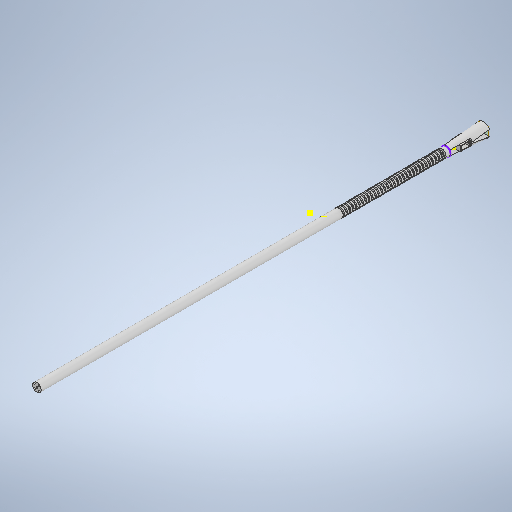
# Autodesk Inventor part: Tool 1
Saved by Autodesk Inventor 2025.2 (Build 292293000, 293)
## iProperties
Created: 2025-03-11
Part Number: Tool 1
Material: Generic
Document SubType Name: Modeling
Designer: avnr2
Density: 1 g/cm^3
Appearance: Default
Author: avnr2
Autodesk Inventor part; units mm, degrees
sketch "Sketch1" plane through (0, 0, 0) normal (0, 1, 0) x (-1, 0, 0)
  circle A0 centre (0, 0) radius 1.5
  dimension "d0" = 3
  constraints: 1 centre point, 1 coincident
  measures "d0" diameter of A0
extrude "Extrusion1" add sketch "Sketch1" along normal blind 40
ref_plane "Work Plane1" through (-40, 0, 0) normal (1, 0, 0) x (0, 1, 0)
sketch "Sketch2" plane through (-40, 0, 0) normal (1, 0, 0) x (0, 1, 0)
  line L0 (0, -1.5) -> (40, -1.5) projected
  line L1 (39.7, -1.5) -> (39.2, -1.5)
  line L2 (39.2, -1.5) -> (39.2, -0.2)
  line L3 (39.2, -0.2) -> (39.7, -0.2)
  line L4 (39.7, -0.2) -> (39.7, -1.5)
  line L5 (38.6, -1.5) -> (38.1, -1.5)
  line L6 (38.1, -1.5) -> (38.1, -0.2)
  line L7 (38.1, -0.2) -> (38.6, -0.2)
  line L8 (38.6, -0.2) -> (38.6, -1.5)
  line L9 (40, -1.5) -> (40, 1.5) projected
  line L10 (40, 0) -> (0, 0)
  line L11 (39.7, 1.5) -> (39.2, 1.5)
  line L12 (39.2, 1.5) -> (39.2, 0.2)
  line L13 (39.2, 0.2) -> (39.7, 0.2)
  line L14 (39.7, 0.2) -> (39.7, 1.5)
  line L15 (38.6, 1.5) -> (38.1, 1.5)
  line L16 (38.1, 1.5) -> (38.1, 0.2)
  line L17 (38.1, 0.2) -> (38.6, 0.2)
  line L18 (38.6, 0.2) -> (38.6, 1.5)
  line L19 (37.8, -1.5) -> (37.8, 1.5)
  line L20 (0, 1.5) -> (40, 1.5) projected
  line L21 (35.9, -1.5) -> (36.4, -1.5)
  line L22 (36.4, -1.5) -> (36.4, -0.2)
  line L23 (36.4, -0.2) -> (35.9, -0.2)
  line L24 (35.9, -0.2) -> (35.9, -1.5)
  line L25 (37, -1.5) -> (37.5, -1.5)
  line L26 (37.5, -1.5) -> (37.5, -0.2)
  line L27 (37.5, -0.2) -> (37, -0.2)
  line L28 (37, -0.2) -> (37, -1.5)
  line L29 (35.9, 1.5) -> (36.4, 1.5)
  line L30 (36.4, 1.5) -> (36.4, 0.2)
  line L31 (36.4, 0.2) -> (35.9, 0.2)
  line L32 (35.9, 0.2) -> (35.9, 1.5)
  line L33 (37, 1.5) -> (37.5, 1.5)
  line L34 (37.5, 1.5) -> (37.5, 0.2)
  line L35 (37.5, 0.2) -> (37, 0.2)
  line L36 (37, 0.2) -> (37, 1.5)
  line L37 (35.6, 1.5) -> (35.6, -1.5)
  line L38 (31.5, -1.5) -> (32, -1.5)
  line L39 (32, -1.5) -> (32, -0.2)
  line L40 (32, -0.2) -> (31.5, -0.2)
  line L41 (31.5, -0.2) -> (31.5, -1.5)
  line L42 (32.6, -1.5) -> (33.1, -1.5)
  line L43 (33.1, -1.5) -> (33.1, -0.2)
  line L44 (33.1, -0.2) -> (32.6, -0.2)
  line L45 (32.6, -0.2) -> (32.6, -1.5)
  line L46 (31.5, 1.5) -> (32, 1.5)
  line L47 (32, 1.5) -> (32, 0.2)
  line L48 (32, 0.2) -> (31.5, 0.2)
  line L49 (31.5, 0.2) -> (31.5, 1.5)
  line L50 (32.6, 1.5) -> (33.1, 1.5)
  line L51 (33.1, 1.5) -> (33.1, 0.2)
  line L52 (33.1, 0.2) -> (32.6, 0.2)
  line L53 (32.6, 0.2) -> (32.6, 1.5)
  line L54 (33.4, -1.5) -> (33.4, 1.5)
  line L55 (35.3, -1.5) -> (34.8, -1.5)
  line L56 (35.3, -0.2) -> (35.3, -1.5)
  line L57 (34.8, -1.5) -> (34.8, -0.2)
  line L58 (34.2, -1.5) -> (33.7, -1.5)
  line L59 (34.2, -0.2) -> (34.2, -1.5)
  line L60 (33.7, -1.5) -> (33.7, -0.2)
  line L61 (33.7, -0.2) -> (34.2, -0.2)
  line L62 (33.7, 0.2) -> (34.2, 0.2)
  line L63 (35.3, 0.2) -> (35.3, 1.5)
  line L64 (34.2, 0.2) -> (34.2, 1.5)
  line L65 (33.7, 1.5) -> (33.7, 0.2)
  line L66 (34.2, 1.5) -> (33.7, 1.5)
  line L67 (34.8, 1.5) -> (34.8, 0.2)
  line L68 (34.8, 0.2) -> (35.3, 0.2)
  line L69 (34.8, -0.2) -> (35.3, -0.2)
  line L70 (35.3, 1.5) -> (34.8, 1.5)
  line L71 (31.2, 1.5) -> (31.2, -1.5)
  line L72 (22.7, -1.5) -> (23.2, -1.5)
  line L73 (23.2, -1.5) -> (23.2, -0.2)
  line L74 (23.2, -0.2) -> (22.7, -0.2)
  line L75 (22.7, -0.2) -> (22.7, -1.5)
  line L76 (23.8, -1.5) -> (24.3, -1.5)
  line L77 (24.3, -1.5) -> (24.3, -0.2)
  line L78 (24.3, -0.2) -> (23.8, -0.2)
  line L79 (23.8, -0.2) -> (23.8, -1.5)
  line L80 (22.4, -1.5) -> (22.4, 1.5)
  line L81 (22.7, 1.5) -> (23.2, 1.5)
  line L82 (23.2, 1.5) -> (23.2, 0.2)
  line L83 (23.2, 0.2) -> (22.7, 0.2)
  line L84 (22.7, 0.2) -> (22.7, 1.5)
  line L85 (23.8, 1.5) -> (24.3, 1.5)
  line L86 (24.3, 1.5) -> (24.3, 0.2)
  line L87 (24.3, 0.2) -> (23.8, 0.2)
  line L88 (23.8, 0.2) -> (23.8, 1.5)
  line L89 (24.6, -1.5) -> (24.6, 1.5)
  line L90 (26.5, -1.5) -> (26, -1.5)
  line L91 (26.5, -0.2) -> (26.5, -1.5)
  line L92 (26, -1.5) -> (26, -0.2)
  line L93 (25.4, -1.5) -> (24.9, -1.5)
  line L94 (25.4, -0.2) -> (25.4, -1.5)
  line L95 (24.9, -1.5) -> (24.9, -0.2)
  line L96 (24.9, -0.2) -> (25.4, -0.2)
  line L97 (24.9, 0.2) -> (25.4, 0.2)
  line L98 (26.5, 0.2) -> (26.5, 1.5)
  line L99 (25.4, 0.2) -> (25.4, 1.5)
  line L100 (24.9, 1.5) -> (24.9, 0.2)
  line L101 (25.4, 1.5) -> (24.9, 1.5)
  line L102 (26, 1.5) -> (26, 0.2)
  line L103 (26, 0.2) -> (26.5, 0.2)
  line L104 (26, -0.2) -> (26.5, -0.2)
  line L105 (26.5, 1.5) -> (26, 1.5)
  line L106 (26.8, 1.5) -> (26.8, -1.5)
  line L107 (30.9, -1.5) -> (30.4, -1.5)
  line L108 (29.3, -1.5) -> (29.3, -0.2)
  line L109 (29.8, -1.5) -> (29.3, -1.5)
  line L110 (29.8, -0.2) -> (29.8, -1.5)
  line L111 (30.4, -1.5) -> (30.4, -0.2)
  line L112 (30.9, -0.2) -> (30.9, -1.5)
  line L113 (29.3, 1.5) -> (29.3, 0.2)
  line L114 (29.3, -0.2) -> (29.8, -0.2)
  line L115 (30.9, 1.5) -> (30.4, 1.5)
  line L116 (30.4, 0.2) -> (30.9, 0.2)
  line L117 (30.4, -0.2) -> (30.9, -0.2)
  line L118 (29, -1.5) -> (29, 1.5)
  line L119 (28.7, 1.5) -> (28.7, 0.2)
  line L120 (28.2, 0.2) -> (28.2, 1.5)
  line L121 (28.7, 0.2) -> (28.2, 0.2)
  line L122 (27.6, 1.5) -> (27.6, 0.2)
  line L123 (27.1, 0.2) -> (27.1, 1.5)
  line L124 (27.6, 0.2) -> (27.1, 0.2)
  line L125 (27.1, 1.5) -> (27.6, 1.5)
  line L126 (28.2, 1.5) -> (28.7, 1.5)
  line L127 (30.9, 0.2) -> (30.9, 1.5)
  line L128 (30.4, 1.5) -> (30.4, 0.2)
  line L129 (29.8, 1.5) -> (29.3, 1.5)
  line L130 (29.3, 0.2) -> (29.8, 0.2)
  line L131 (29.8, 0.2) -> (29.8, 1.5)
  line L132 (27.6, -0.2) -> (27.1, -0.2)
  line L133 (28.7, -0.2) -> (28.2, -0.2)
  line L134 (27.1, -1.5) -> (27.6, -1.5)
  line L135 (27.1, -0.2) -> (27.1, -1.5)
  line L136 (27.6, -1.5) -> (27.6, -0.2)
  line L137 (28.2, -0.2) -> (28.2, -1.5)
  line L138 (28.7, -1.5) -> (28.7, -0.2)
  line L139 (28.2, -1.5) -> (28.7, -1.5)
  line L140 (5.1, -1.5) -> (5.6, -1.5)
  line L141 (5.6, -1.5) -> (5.6, -0.2)
  line L142 (5.6, -0.2) -> (5.1, -0.2)
  line L143 (5.1, -0.2) -> (5.1, -1.5)
  line L144 (6.2, -1.5) -> (6.7, -1.5)
  line L145 (6.7, -1.5) -> (6.7, -0.2)
  line L146 (6.7, -0.2) -> (6.2, -0.2)
  line L147 (6.2, -0.2) -> (6.2, -1.5)
  line L148 (4.8, -1.5) -> (4.8, 1.5)
  line L149 (5.1, 1.5) -> (5.6, 1.5)
  line L150 (5.6, 1.5) -> (5.6, 0.2)
  line L151 (5.6, 0.2) -> (5.1, 0.2)
  line L152 (5.1, 0.2) -> (5.1, 1.5)
  line L153 (6.2, 1.5) -> (6.7, 1.5)
  line L154 (6.7, 1.5) -> (6.7, 0.2)
  line L155 (6.7, 0.2) -> (6.2, 0.2)
  line L156 (6.2, 0.2) -> (6.2, 1.5)
  line L157 (7, -1.5) -> (7, 1.5)
  line L158 (8.9, -1.5) -> (8.4, -1.5)
  line L159 (8.9, -0.2) -> (8.9, -1.5)
  line L160 (8.4, -1.5) -> (8.4, -0.2)
  line L161 (7.8, -1.5) -> (7.3, -1.5)
  line L162 (7.8, -0.2) -> (7.8, -1.5)
  line L163 (7.3, -1.5) -> (7.3, -0.2)
  line L164 (7.3, -0.2) -> (7.8, -0.2)
  line L165 (7.3, 0.2) -> (7.8, 0.2)
  line L166 (8.9, 0.2) -> (8.9, 1.5)
  line L167 (7.8, 0.2) -> (7.8, 1.5)
  line L168 (7.3, 1.5) -> (7.3, 0.2)
  line L169 (7.8, 1.5) -> (7.3, 1.5)
  line L170 (8.4, 1.5) -> (8.4, 0.2)
  line L171 (8.4, 0.2) -> (8.9, 0.2)
  line L172 (8.4, -0.2) -> (8.9, -0.2)
  line L173 (8.9, 1.5) -> (8.4, 1.5)
  line L174 (9.2, 1.5) -> (9.2, -1.5)
  line L175 (13.3, -1.5) -> (12.8, -1.5)
  line L176 (11.7, -1.5) -> (11.7, -0.2)
  line L177 (12.2, -1.5) -> (11.7, -1.5)
  line L178 (12.2, -0.2) -> (12.2, -1.5)
  line L179 (12.8, -1.5) -> (12.8, -0.2)
  line L180 (13.3, -0.2) -> (13.3, -1.5)
  line L181 (11.7, 1.5) -> (11.7, 0.2)
  line L182 (11.7, -0.2) -> (12.2, -0.2)
  line L183 (13.3, 1.5) -> (12.8, 1.5)
  line L184 (12.8, 0.2) -> (13.3, 0.2)
  line L185 (12.8, -0.2) -> (13.3, -0.2)
  line L186 (11.4, -1.5) -> (11.4, 1.5)
  line L187 (11.1, 1.5) -> (11.1, 0.2)
  line L188 (10.6, 0.2) -> (10.6, 1.5)
  line L189 (11.1, 0.2) -> (10.6, 0.2)
  line L190 (10, 1.5) -> (10, 0.2)
  line L191 (9.5, 0.2) -> (9.5, 1.5)
  line L192 (10, 0.2) -> (9.5, 0.2)
  line L193 (9.5, 1.5) -> (10, 1.5)
  line L194 (10.6, 1.5) -> (11.1, 1.5)
  line L195 (13.3, 0.2) -> (13.3, 1.5)
  line L196 (12.8, 1.5) -> (12.8, 0.2)
  line L197 (12.2, 1.5) -> (11.7, 1.5)
  line L198 (11.7, 0.2) -> (12.2, 0.2)
  line L199 (12.2, 0.2) -> (12.2, 1.5)
  line L200 (10, -0.2) -> (9.5, -0.2)
  line L201 (11.1, -0.2) -> (10.6, -0.2)
  line L202 (9.5, -1.5) -> (10, -1.5)
  line L203 (9.5, -0.2) -> (9.5, -1.5)
  line L204 (10, -1.5) -> (10, -0.2)
  line L205 (10.6, -0.2) -> (10.6, -1.5)
  line L206 (11.1, -1.5) -> (11.1, -0.2)
  line L207 (10.6, -1.5) -> (11.1, -1.5)
  line L208 (13.6, 1.5) -> (13.6, -1.5)
  line L209 (21.6, -0.2) -> (22.1, -0.2)
  line L210 (20.5, -0.2) -> (21, -0.2)
  line L211 (22.1, 1.5) -> (21.6, 1.5)
  line L212 (22.1, -1.5) -> (21.6, -1.5)
  line L213 (21.6, -1.5) -> (21.6, -0.2)
  line L214 (22.1, -0.2) -> (22.1, -1.5)
  line L215 (21, -0.2) -> (21, -1.5)
  line L216 (20.5, -1.5) -> (20.5, -0.2)
  line L217 (21, -1.5) -> (20.5, -1.5)
  line L218 (15.8, -1.5) -> (15.8, 1.5)
  line L219 (15, 0.2) -> (15, 1.5)
  line L220 (15, 1.5) -> (15.5, 1.5)
  line L221 (15.5, 0.2) -> (15, 0.2)
  line L222 (14.4, 1.5) -> (14.4, 0.2)
  line L223 (13.9, 0.2) -> (13.9, 1.5)
  line L224 (13.9, 1.5) -> (14.4, 1.5)
  line L225 (14.4, 0.2) -> (13.9, 0.2)
  line L226 (15.5, 1.5) -> (15.5, 0.2)
  line L227 (20.2, -1.5) -> (20.2, 1.5)
  line L228 (20.5, 1.5) -> (20.5, 0.2)
  line L229 (21, 1.5) -> (20.5, 1.5)
  line L230 (20.5, 0.2) -> (21, 0.2)
  line L231 (21, 0.2) -> (21, 1.5)
  line L232 (22.1, 0.2) -> (22.1, 1.5)
  line L233 (21.6, 0.2) -> (22.1, 0.2)
  line L234 (21.6, 1.5) -> (21.6, 0.2)
  line L235 (19.9, 1.5) -> (19.9, 0.2)
  line L236 (19.9, 0.2) -> (19.4, 0.2)
  line L237 (19.4, 0.2) -> (19.4, 1.5)
  line L238 (18.3, 1.5) -> (18.8, 1.5)
  line L239 (18.8, 1.5) -> (18.8, 0.2)
  line L240 (19.9, -0.2) -> (19.4, -0.2)
  line L241 (18.3, 0.2) -> (18.3, 1.5)
  line L242 (18.8, 0.2) -> (18.3, 0.2)
  line L243 (18, 1.5) -> (18, -1.5)
  line L244 (18.8, -0.2) -> (18.3, -0.2)
  line L245 (18.3, -1.5) -> (18.8, -1.5)
  line L246 (18.3, -0.2) -> (18.3, -1.5)
  line L247 (18.8, -1.5) -> (18.8, -0.2)
  line L248 (19.4, -0.2) -> (19.4, -1.5)
  line L249 (19.4, -1.5) -> (19.9, -1.5)
  line L250 (19.9, -1.5) -> (19.9, -0.2)
  line L251 (19.4, 1.5) -> (19.9, 1.5)
  line L252 (13.9, -1.5) -> (14.4, -1.5)
  line L253 (14.4, -0.2) -> (13.9, -0.2)
  line L254 (15.5, -0.2) -> (15, -0.2)
  line L255 (15.5, -1.5) -> (15.5, -0.2)
  line L256 (15, -1.5) -> (15.5, -1.5)
  line L257 (15, -0.2) -> (15, -1.5)
  line L258 (14.4, -1.5) -> (14.4, -0.2)
  line L259 (13.9, -0.2) -> (13.9, -1.5)
  line L260 (17.2, 0.2) -> (17.7, 0.2)
  line L261 (17.7, 0.2) -> (17.7, 1.5)
  line L262 (17.7, 1.5) -> (17.2, 1.5)
  line L263 (17.2, 1.5) -> (17.2, 0.2)
  line L264 (16.6, 0.2) -> (16.6, 1.5)
  line L265 (16.1, 1.5) -> (16.1, 0.2)
  line L266 (16.6, 1.5) -> (16.1, 1.5)
  line L267 (16.1, 0.2) -> (16.6, 0.2)
  line L268 (17.2, -0.2) -> (17.7, -0.2)
  line L269 (17.7, -0.2) -> (17.7, -1.5)
  line L270 (17.7, -1.5) -> (17.2, -1.5)
  line L271 (17.2, -1.5) -> (17.2, -0.2)
  line L272 (16.1, -0.2) -> (16.6, -0.2)
  line L273 (16.1, -1.5) -> (16.1, -0.2)
  line L274 (16.6, -1.5) -> (16.1, -1.5)
  line L275 (16.6, -0.2) -> (16.6, -1.5)
  point P0 (22.4, 0)
  point P1 (4.8, 0)
  dimension "d4" = 1.3
  dimension "d5" = 0.5
  dimension "d6" = 0.5
  dimension "d7" = 0.6
  dimension "d8" = 40
  dimension "d9" = 0.3
  dimension "d10" = 0.3
  dimension "d11" = 0.3
  dimension "d12" = 0.3
  constraints: 546 end point, 278 symmetric about line, 4 parallel, 3 perpendicular, 3 vertical, 2 horizontal, 1 midpoint, 10 other
  measures "d4" distance of L3.end L1.start
  measures "d5" distance of L2.end L3.end
  measures "d6" distance of L6.end L7.end
  measures "d7" distance between parallel lines of L8 L2
  measures "d8" distance of L10.start L10.end
  measures "d9" distance between parallel lines of L19 L6
  measures "d10" distance between parallel lines of L37 L24
  measures "d11" distance between parallel lines of L41 L71
  measures "d12" distance between parallel lines of L75 L80
extrude "Extrusion2" cut sketch "Sketch2" along normal blind 54.75 and the other way blind 5 contours L143 L142 L141 L0 | L147 L146 L145 L0 | L20 L150 L151 L152 | L163 L164 L162 L0 | L154 L155 L156 L20 | L20 L167 L165 L168 | L166 L171 L170 L20 | L20 L190 L192 L191 | L0 L160 L172 L159 | L203 L200 L204 L0 | L0 L205 L201 L206 | L176 L182 L178 L0 | L187 L189 L188 L20 | L20 L199 L198 L181 | L195 L184 L196 L20 | L20 L222 L225 L223 | L0 L179 L185 L180 | L259 L253 L258 L0 | L0 L257 L254 L255 | L273 L272 L275 L0 | L226 L221 L219 L20 | L20 L264 L267 L265 | L261 L260 L263 L20 | L20 L239 L242 L241 | L0 L271 L268 L269 | L246 L244 L247 L0 | L0 L248 L240 L250 | L216 L210 L215 L0 | L235 L236 L237 L20 | L20 L231 L230 L228 | L0 L213 L209 L214 | L75 L74 L73 L0 | L232 L233 L234 L20 | L20 L82 L83 L84 | L0 L79 L78 L77 | L95 L96 L94 L0 | L86 L87 L88 L20 | L20 L99 L97 L100 | L98 L103 L102 L20 | L20 L122 L124 L123 | L0 L92 L104 L91 | L135 L132 L136 L0 | L0 L137 L133 L138 | L108 L114 L110 L0 | L119 L121 L120 L20 | L20 L131 L130 L113 | L127 L116 L128 L20 | L20 L47 L48 L49 | L0 L111 L117 L112 | L41 L40 L39 L0 | L0 L45 L44 L43 | L60 L61 L59 L0 | L51 L52 L53 L20 | L20 L64 L62 L65 | L63 L68 L67 L20 | L20 L30 L31 L32 | L0 L57 L69 L56 | L24 L23 L22 L0 | L0 L28 L27 L26 | L6 L7 L8 L0 | L34 L35 L36 L20 | L15 L18 L17 L16 | L0 L2 L3 L4 | L14 L13 L12 L11
sketch "Sketch3" plane through (0, 0, 0) normal (0, -1, 0) x (1, 0, 0)
  circle A0 centre (0, 0) radius 0.3
  dimension "d17" = 0.6
  constraints: 1 centre point, 1 coincident
  measures "d17" diameter of A0
extrude "Extrusion3" cut sketch "Sketch3" against normal blind 54.75
sketch "Sketch4" plane through (0, 0, 0) normal (0, -1, 0) x (1, 0, 0)
  circle A0 centre (0, 0) radius 1.15 construction
  circle A1 centre (-0.7909, -0.8348) radius 0.3
  circle A2 centre (0, 0) radius 1.15 construction
  circle A3 centre (0.8348, -0.7909) radius 0.3
  circle A4 centre (0, 0) radius 1.15 construction
  circle A5 centre (0.7909, 0.8348) radius 0.3
  circle A6 centre (0, 0) radius 1.15 construction
  circle A7 centre (-0.8348, 0.7909) radius 0.3
  dimension "d23" = 2.3
  dimension "d22" = 0.6
  dimension "d26" = 360
  constraints: 6 coincident, 4 centre point, 31 other
  measures "d22" diameter of A1
extrude "Extrusion4" cut sketch "Sketch4" against normal blind 54.75
sketch "Sketch5" plane through (0, 40, 0) normal (0, 1, 0) x (1, 0, 0)
  point P0 (0, 0)
sketch "Sketch6" plane through (0, 40, 0) normal (0, 1, 0) x (1, 0, 0)
  circle A0 centre (0, 0) radius 0.3 projected
  circle A1 centre (0, 0) radius 0.7513
  constraints: 1 centre point, 1 coincident
extrude "Extrusion5" add sketch "Sketch6" along normal blind 0.6
sketch "Sketch7" plane through (0, 40.6, 0) normal (0, 1, 0) x (1, 0, 0)
  circle A0 centre (0, 0) radius 1.5
  constraints: 1 centre point, 1 coincident
extrude "Extrusion6" add sketch "Sketch7" along normal blind 0.6
sketch "Sketch8" plane through (0, 41.2, 0) normal (0, 1, 0) x (1, 0, 0)
  circle A0 centre (0, 0) radius 0.3 projected
  circle A1 centre (0, 0) radius 0.3
  constraints: 1 centre point, 1 coincident
extrude "Extrusion7" cut sketch "Sketch8" against normal blind 0.6
sketch "Sketch9" plane through (0, 41.2, 0) normal (0, 1, 0) x (1, 0, 0)
  circle A0 centre (0, 0) radius 1.5
  constraints: 1 centre point, 1 coincident
extrude "Extrusion8" add sketch "Sketch9" along normal blind 10
ref_plane "Work Plane2" through (-13.25, 0, 0) normal (1, 0, 0) x (0, 1, 0)
sketch "Sketch10" plane through (-13.25, 0, 0) normal (1, 0, 0) x (0, 1, 0)
  line L0 (51.2, -1.5) -> (51.2, 1.5) projected
  line L1 (51.2, 0) -> (42.026, 0)
  line L2 (51.2, 0.05) -> (47.2, 0.05)
  line L3 (47.2, 0.05) -> (47.2, -0.05)
  line L4 (47.2, -0.05) -> (51.2, -0.05)
  line L5 (51.2, -0.05) -> (51.2, 0.05)
  line L6 (51.2, 0.05) -> (47.2, -0.05) construction
  line L7 (47.2, 0.05) -> (51.2, -0.05) construction
  point P0 (0, 0)
  point P1 (49.2, 0)
  dimension "d39" = 4
  dimension "d40" = 0.1
  constraints: 14 end point, 4 midpoint, 2 horizontal, 2 parallel, 1 perpendicular, 1 point on line
  measures "d39" distance of L3.end L4.end
  measures "d40" distance of L2.end L3.end
extrude "Extrusion9" cut sketch "Sketch10" along normal blind 20.75
sketch "Sketch11" plane through (-13.25, 0, 0) normal (1, 0, 0) x (0, 1, 0)
  line L0 (47.2, 0.05) -> (51.2, 0.05) projected
  line L1 (47.2, 0.05) -> (47, 0.05)
  line L2 (47, 0.05) -> (47, 0.55)
  line L3 (47, 0.55) -> (45, 0.55)
  line L4 (45, -0.5) -> (47, -0.5)
  line L5 (47, -0.5) -> (47, -0.05)
  line L6 (47.2, -0.05) -> (51.2, -0.05) projected
  line L7 (47, -0.05) -> (47.2, -0.05)
  line L8 (47.2, -0.05) -> (47.2, -0.3)
  line L9 (47.2, -0.3) -> (47.1, -0.3)
  line L10 (47.1, -0.3) -> (47.1, -0.7)
  line L11 (47.1, -0.7) -> (44.6, -0.7)
  line L12 (44.6, 0.75) -> (47.1, 0.75)
  line L13 (47.1, 0.75) -> (47.1, 0.3)
  line L14 (47.1, 0.3) -> (47.2, 0.3)
  line L15 (47.2, 0.3) -> (47.2, 0.05)
  line L16 (47.2, 0.05) -> (47.2, -0.05) projected
  line L17 (47.2, 0) -> (44.6089, 0)
  line L18 (45, 0.55) -> (45, -0.5)
  line L19 (44.6, 0.75) -> (44.6, -0.7)
  line L20 (47.2, 0.3) -> (47.2, 1)
  line L21 (47.2, 1) -> (41.9867, 1)
  line L22 (47.2, -0.3) -> (47.2, -1)
  line L23 (47.2, -1) -> (41.9867, -1)
  line L24 (40.6, -1.5) -> (51.2, -1.5) projected
  line L25 (41.9867, -1) -> (41.9867, 1)
  point P0 (0, 0)
  dimension "d43" = 0.2
  dimension "d44" = 0.5
  dimension "d45" = 2
  dimension "d48" = 0.25
  dimension "d51" = 0.75
  dimension "d52" = 0.2
  dimension "d53" = 0.2
  dimension "d54" = 2.5911
  dimension "d55" = 0.5
  dimension "d56" = 0.1
  dimension "d57" = 0.2
  dimension "d58" = 0.25
  dimension "d59" = 2.5
  dimension "d60" = 2.5
  dimension "d67" = 1
  dimension "d68" = 1
  constraints: 44 end point, 11 perpendicular, 6 horizontal alignment, 6 vertical alignment, 4 point on line, 3 parallel, 2 horizontal, 2 vertical, 1 midpoint
  measures "d43" distance of L0.start L1.end
  measures "d44" distance of L1.end L2.end
  measures "d45" distance of L2.end L3.end
  measures "d48" distance of L14.end L0.start
  measures "d51" distance between parallel lines of L17 L12
  measures "d52" distance between parallel lines of L3 L12
  measures "d53" distance between parallel lines of L11 L4
  measures "d54" distance of L17.start L17.end
  measures "d55" distance between parallel lines of L4 L17
  measures "d56" distance of L8.end L9.end
  measures "d57" distance between parallel lines of L5 L8
  measures "d58" distance between parallel lines of L9 L7
  measures "d59" distance of L10.end L11.end
  measures "d60" distance of L12.start L12.end
  measures "d67" distance between parallel lines of L17 L21
  measures "d68" distance between parallel lines of L17 L23
extrude "Extrusion10" cut sketch "Sketch11" along normal blind 20.754 contours L16 L17 L18 L3 L2 L1 | L14 L13 L12 L19 L11 L10 L9 L22 L23 L25 L21 L20 | L16 L7 L5 L4 L18 L17
sketch "Sketch12" plane through (-1.3266, 44.6, -0.7) normal (0, -1, 0) x (1, 0, 0)
  point P0 (1.3266, 0.7)
sketch "Sketch13" plane through (-1.118, 41.9867, 1) normal (0, 1, 0) x (1, 0, 0)
  point P0 (1.118, 1)
sketch "Sketch14" plane through (0, 0, 0) normal (0, -1, 0) x (1, 0, 0)
  circle A0 centre (0, 0) radius 0.3
  constraints: 1 centre point, 1 coincident
extrude "Extrusion11" cut sketch "Sketch14" against normal blind 46.004
sketch "Sketch16" plane through (-1.299, 44.6, 0.75) normal (0, 0, 1) x (1, 0, 0)
  point P0 (1.299, -44.6)
sketch "Sketch17" plane through (0, 40.6, 0) normal (0, -1, 0) x (1, 0, 0)
  circle A0 centre (0, 0) radius 0.3
  circle A1 centre (0.8348, -0.7909) radius 0.3 projected
  circle A2 centre (0.8348, -0.7909) radius 0.3
  circle A3 centre (-0.7909, -0.8348) radius 0.3 projected
  circle A4 centre (-0.7909, -0.8348) radius 0.3
  circle A5 centre (-0.8348, 0.7909) radius 0.3 projected
  circle A6 centre (-0.8348, 0.7909) radius 0.3
  circle A7 centre (0.7909, 0.8348) radius 0.3 projected
  circle A8 centre (0.7909, 0.8348) radius 0.3
  circle A9 centre (0, 0) radius 0.3
  circle A10 centre (0, 0) radius 1.5
  constraints: 7 centre point, 7 coincident, 1 concentric
sketch "Sketch18" plane through (0, 0, 0) normal (0, -1, 0) x (1, 0, 0)
  point P0 (0, 0)
sketch "Sketch19" plane through (0, 0, 0) normal (0, -1, 0) x (1, 0, 0)
  arc A0 (-0.2236, -0.2) -> (0.2236, -0.2) centre (0, 0) ccw projected
  circle A1 centre (0, 0) radius 0.3
  circle A2 centre (-0.7892, -0.8405) radius 0.2991
  circle A3 centre (-0.8354, 0.7848) radius 0.2954
  circle A4 centre (0.7909, 0.8348) radius 0.3 projected
  circle A5 centre (0.7909, 0.8348) radius 0.3
  circle A6 centre (0.8348, -0.7909) radius 0.3 projected
  circle A7 centre (0.8348, -0.7909) radius 0.3
  circle A8 centre (0, 0) radius 1.5
  constraints: 6 centre point, 4 coincident
extrude "Extrusion13" add sketch "Sketch19" along normal blind 99
sketch "Sketch21" plane through (0, 51.2, 0) normal (0, 1, 0) x (1, 0, 0)
  circle A0 centre (0, 0) radius 1.5
  constraints: 1 centre point, 1 coincident
extrude "Extrusion14" cut sketch "Sketch21" against normal blind 4
extrude "Extrusion18" cut sketch "Sketch17" against normal blind 8 contours A0 | A1 | A3 | A5 | A7 | A10
sketch "Sketch36" plane through (0, 40.6, 0) normal (0, 1, 0) x (1, 0, 0)
  circle A0 centre (0, 0) radius 1.5
  constraints: 1 centre point, 1 coincident
extrude "Extrusion19" add sketch "Sketch36" along normal blind 1.5
sketch "Sketch37" plane through (0, 42.1, 0) normal (0, 1, 0) x (1, 0, 0)
  circle A0 centre (0, 0) radius 0.3
  dimension "d97" = 0.6
  constraints: 1 centre point, 1 coincident
  measures "d97" diameter of A0
extrude "Extrusion20" cut sketch "Sketch37" against normal blind 1.5
ref_plane "Work Plane3" through (0, 55, 0) normal (0, 1, 0) x (-1, 0, 0)
sketch "Sketch38" plane through (0, 55, 0) normal (0, 1, 0) x (-1, 0, 0)
  arc A0 (-0.2236, -0.2) -> (0.2236, -0.2) centre (0, 0) ccw projected
  circle A1 centre (0, 0) radius 2.375
  dimension "d101" = 4.75
  constraints: 1 centre point, 1 coincident
  measures "d101" diameter of A1
sketch "Sketch39" plane through (0, 42.1, 0) normal (0, 1, 0) x (1, 0, 0)
  circle A0 centre (0, 0) radius 1.5
  constraints: 1 centre point, 1 coincident
loft "Loft3" add profiles "Sketch38" section 1 edges at (-1.5, 42.1, 0)
ref_plane "Work Plane4" through (-5, 0, 0) normal (1, 0, 0) x (0, 1, 0)
sketch "Sketch40" plane through (-5, 0, 0) normal (1, 0, 0) x (0, 1, 0)
  line L0 (55, 2.375) -> (55, -2.375) projected
  line L1 (55, 1.125) -> (55, -1.125)
  line L2 (48, 2.5762) -> (48, -2.6905)
  line L3 (48, 0) -> (55, 1.125)
  line L4 (48, 0) -> (55, -1.125)
  point P0 (0, 0)
  point P1 (55, 0)
  dimension "d107" = 2.25
  dimension "d108" = 7
  constraints: 8 end point, 3 point on line, 2 midpoint, 1 vertical
  measures "d107" distance of L1.start L1.end
  measures "d108" distance between parallel lines of L2 L0
extrude "Extrusion21" cut sketch "Sketch40" along normal blind 13.75
sketch "Sketch43" plane through (-5, 0, 0) normal (1, 0, 0) x (0, 1, 0)
  line L0 (55, 1.125) -> (48, 0) projected
  line L1 (49.0674, 0.1715) -> (48.9013, 1.2052)
  line L2 (48.9013, 1.2052) -> (42.9484, 0.93)
  line L3 (42.9913, 0) -> (49.095, 0)
  line L4 (42.9484, 0.93) -> (42.1, 0.8908)
  line L5 (42.1, -1.5) -> (42.1, 1.5) projected
  line L6 (42.1, 0) -> (42.9913, 0)
  point P0 (0, 0)
  constraints: 10 end point, 2 perpendicular, 2 point on line, 1 horizontal, 1 midpoint
sketch "Sketch44" plane through (-5, 0, 0) normal (1, 0, 0) x (0, 1, 0)
  line L0 (55, 1.125) -> (48, 0) projected
  line L1 (49.067, 0.1715) -> (49.0945, 0)
  line L2 (49.0945, 0) -> (42.1, 0)
  line L3 (42.1, 0.3) -> (42.1, -0.3) projected
  line L4 (42.1, -1.5) -> (42.1, 1.5) projected
  line L5 (42.1, 0.8813) -> (48.9003, 1.2082)
  line L6 (48.9003, 1.2082) -> (49.067, 0.1715)
  line L7 (49.067, -0.1715) -> (49.0945, 0)
  line L8 (42.1, -0.3) -> (42.1, 0.3)
  line L9 (42.1, -0.8813) -> (48.9003, -1.2082)
  line L10 (48.9003, -1.2082) -> (49.067, -0.1715)
  line L11 (49.067, 0.1715) -> (48.9003, 0.1447)
  line L12 (48.9003, 0.1447) -> (48.8775, 0.2871)
  line L13 (48.8775, 0.2871) -> (49.0441, 0.3138)
  line L14 (48.8775, 0.2871) -> (48.782, 0.8813)
  line L15 (48.782, 0.8813) -> (46.3641, 0.7651)
  line L16 (46.3641, 0.7651) -> (46.4341, -0.69)
  point P0 (0, 0)
  point P1 (48, 0)
  point P2 (48, 0)
  constraints: 28 end point, 6 point on line, 6 symmetric about line, 3 perpendicular, 1 collinear, 1 midpoint, 1 parallel
extrude "Extrusion23" cut sketch "Sketch44" along normal blind 100 contours L0 L12 L13 L6 | L0 L2 L16 L15 L14 L12 | L7 L10 L9 L4 L3 L2 | L13 L14 L15 L16 L2 L3 L4 L5 L6
sketch "Sketch48" plane through (-5, 0, 0) normal (1, 0, 0) x (0, 1, 0)
  point P0 (0, 0)
sketch "Sketch49" plane through (-5, 0, 0) normal (1, 0, 0) x (0, 1, 0)
  point P0 (0, 0)
ref_plane "Work Plane5" through (-1.75, 0, 0) normal (1, 0, 0) x (0, 1, 0)
sketch "Sketch50" plane through (-1.75, 0, 0) normal (1, 0, 0) x (0, 1, 0)
  line L0 (55, 1.125) -> (49.067, 0.1715) projected
  line L1 (51.1226, 0.5019) -> (48, 0)
  line L2 (48, 0) -> (49.9534, -0.3139)
  line L3 (49.067, -0.1715) -> (55, -1.125) projected
  line L4 (49.067, 0.1715) -> (48.7708, 0.1239)
  line L5 (48.7708, 0.1239) -> (48.7232, 0.4201)
  line L6 (48.7232, 0.4201) -> (49.0194, 0.4677)
  line L7 (49.0194, 0.4677) -> (49.067, 0.1715)
  line L8 (48.7232, 0.4201) -> (48.6318, 0.9885)
  line L9 (48.6318, 0.9885) -> (45.2206, 0.7661)
  line L10 (45.2206, 0.7661) -> (45.2206, 0)
  line L11 (45.2206, 0) -> (48, 0)
  line L12 (48.6227, 0.1001) -> (48.5133, 0.7803)
  line L13 (48.5133, 0.7803) -> (45.6206, 0.5918)
  line L14 (45.6206, 0.5918) -> (45.6206, 0)
  line L15 (49.067, -0.1715) -> (48.7708, -0.1239)
  line L16 (48.7708, -0.1239) -> (48.7232, -0.4201)
  line L17 (48.7232, -0.4201) -> (49.0194, -0.4677)
  line L18 (49.0194, -0.4677) -> (49.067, -0.1715)
  line L19 (48.7232, -0.4201) -> (48.622, -1.0605)
  line L20 (48.622, -1.0605) -> (45.2206, -0.8495)
  line L21 (45.2206, -0.8495) -> (45.2206, 0)
  line L22 (45.6206, 0) -> (45.6206, -0.674)
  line L23 (45.6206, -0.674) -> (48.4985, -0.8525)
  line L24 (48.6195, -0.0996) -> (48.4985, -0.8525)
  point P0 (0, 0)
  point P1 (48.6726, -0.7403)
  dimension "d134" = 0.3
  dimension "d136" = 0.3
  dimension "d137" = 0.3
  dimension "d138" = 0.3
  dimension "d139" = 0.3
  dimension "d140" = 0.3
  dimension "d141" = 0.15
  dimension "d145" = 0.4
  dimension "d146" = 0.2
  dimension "d147" = 0.2
  dimension "d148" = 3.4079
  dimension "d149" = 0.15
  constraints: 46 end point, 8 point on line, 7 perpendicular, 3 parallel, 3 vertical, 1 collinear, 1 midpoint
  measures "d134" distance of L0.end L4.end
  measures "d136" distance of L5.end L6.end
  measures "d137" distance of L3.start L15.end
  measures "d138" distance of L15.end L16.end
  measures "d139" distance of L16.end L17.end
  measures "d140" distance of L17.end L3.start
  measures "d141" distance between parallel lines of L12 L8
  measures "d145" distance between parallel lines of L10 L14
  measures "d146" distance between parallel lines of L20 L23
  measures "d147" distance between parallel lines of L13 L9
  measures "d148" distance of L19.end L20.end
  measures "d149" angle of L24 L19
extrude "Extrusion24" add sketch "Sketch50" along normal blind 3.5 contours L1 L5 L6 L7 | L1 L12 L13 L14 L11 L10 L9 L8 L5 | L2 L16 L19 L20 L21 L11 L22 L23 L24 | L2 L18 L17 L16
sketch "Sketch51" plane through (0, -99, 0) normal (0, -1, 0) x (1, 0, 0)
  circle A0 centre (0, 0) radius 0.3
  constraints: 1 centre point, 1 coincident
extrude "Extrusion25" cut sketch "Sketch51" against normal blind 145.25
body "Solid1"
